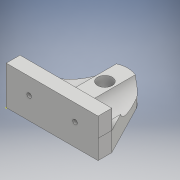
# Autodesk Inventor part: lower_deck_shaft_mount
Saved by Autodesk Inventor 2017 (Build 210142000, 142)
## iProperties
Created: 2017-08-21
Part Number: lower_deck_shaft_mount
Material: Generic
Document SubType Name: Modeling
Designer: ndz
Density: 1 g/cm^3
Appearance: Default
Author: ndz
Autodesk Inventor part; units mm, degrees
ref_plane "YZ Plane" through (0, 0, 0) normal (1, 0, 0) x (0, 1, 0)
ref_plane "XZ Plane" through (0, 0, 0) normal (0, 1, 0) x (-1, 0, 0)
ref_plane "XY Plane" through (0, 0, 0) normal (0, 0, 1) x (1, 0, 0)
sketch "Sketch1" plane through (0, 0, 0) normal (0, 0, 1) x (1, 0, 0)
  circle A0 centre (10, 11.5) radius 1.6
  line L0 (0, 0) -> (20.0001, 0)
  line L1 (0, 0) -> (0, 3)
  line L2 (20.0001, 0) -> (20.0001, 3)
  line L3 (0, 3) -> (16, 3) construction
  line L4 (20.0001, 3) -> (36.0001, 3) construction
  arc A1 (14.3301, 14) -> (5.6699, 14) centre (10, 11.5) ccw
  line L5 (10, 11.5) -> (5.6699, 14) construction
  line L6 (10, 11.5) -> (14.3301, 14) construction
  line L7 (5.6699, 14) -> (0, 3)
  line L8 (14.3301, 14) -> (20.0001, 3)
  dimension "d17" = 3
  dimension "d18" = 3
  dimension "d19" = 11.5
  dimension "d23" = 90
  dimension "d24" = 90
  dimension "d25" = 10
  dimension "d31" = 5
  dimension "d32" = 120
  dimension "d33" = 14
  constraints: 18 end point, 2 centre point, 2 horizontal, 2 point on circle, 1 coincident, 1 vertical
  measures "d17" distance of L0.start L1.end
  measures "d18" distance of L0.end L2.end
  measures "d19" distance from line of A0.centre L0
  measures "d23" angle of L0 L1
  measures "d24" angle of L0 L2
  measures "d25" distance from line of L1 A0.centre
  measures "d31" radius of A1
  measures "d32" angle of L6 L5
  measures "d33" distance from line of L0 L5.end
sketch "Sketch3" plane through (0, 0, 0) normal (0, 0, 1) x (1, 0, 0)
  point P0 (0, 0)
extrude "Extrusion1" add sketch "Sketch1" along normal blind 4.2
sketch "Sketch4" plane through (0, 0, 4.2) normal (0, 0, 1) x (1, 0, 0)
  line L0 (0, 3) -> (0, 0) projected
  line L1 (20.0001, 0) -> (20.0001, 3) projected
  line L2 (0, 0) -> (20.0001, 0)
  line L3 (20.0001, 0) -> (20.0001, 3)
  line L4 (3.884, 22.9404) -> (-0.9789, 3.2417) projected
  line L5 (20.0001, 3) -> (0, 3)
  line L6 (0, 3) -> (0, 0)
  constraints: 8 end point, 3 perpendicular, 1 collinear
extrude "Extrusion2" add sketch "Sketch4" along normal blind 4.2
sketch "Sketch5" plane through (0, 0, 0) normal (0, -1, 0) x (1, 0, 0)
  circle A0 centre (5, 4.8) radius 0.5
  circle A1 centre (15, 4.8) radius 0.5
  line L0 (0, 0) -> (20.0001, 0) projected
  dimension "d13" = 1
  dimension "d14" = 1
  dimension "d38" = 4.8
  dimension "d39" = 4.8
  constraints: 2 centre point
  measures "d13" diameter of A0
  measures "d14" diameter of A1
  measures "d38" distance from line of L0 A0.centre
  measures "d39" distance from line of L0 A1.centre
extrude "Extrusion3" cut sketch "Sketch5" against normal blind 5.5
sketch "Sketch6" plane through (0, 3, 8.4) normal (0, 1, 0) x (1, 0, 0)
  circle A0 centre (5, 3.6) radius 0.5 projected
  circle A1 centre (5, 3.6) radius 3
  circle A2 centre (15, 3.6) radius 0.5 projected
  circle A3 centre (15, 3.6) radius 3
  line L0 (0, 8.4) -> (20.0001, 8.4) projected
  dimension "d34" = 6
  dimension "d35" = 6
  dimension "d40" = 4.8
  dimension "d41" = 4.8
  constraints: 2 centre point, 2 coincident
  measures "d34" diameter of A1
  measures "d35" diameter of A3
  measures "d40" distance from line of L0 A1.centre
  measures "d41" distance from line of L0 A3.centre
extrude "Extrusion4" cut sketch "Sketch6" along normal up to next
body "Solid1"
